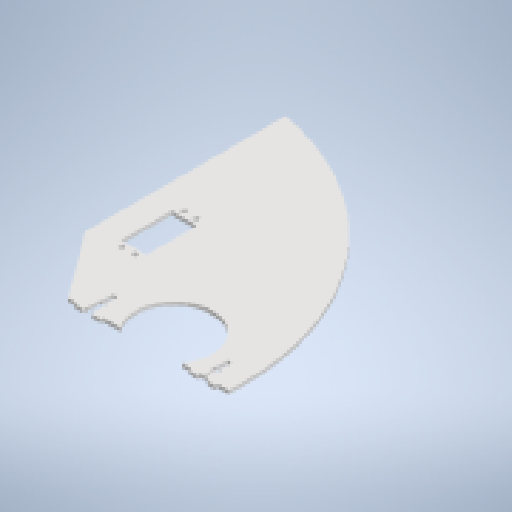
# Autodesk Inventor part: боковые стороны головы
Saved by Autodesk Inventor 2023.2 (Build 272271030, 271C)
## iProperties
Created: 2024-01-31
Part Number: боковые стороны головы
Material: Типовые
Document SubType Name: Modeling
Designer: I9232
Density: 1 g/cm^3
Appearance: По умолчанию
Author: I9232
Autodesk Inventor part; units mm, degrees
ref_plane "YZ Plane" through (0, 0, 0) normal (1, 0, 0) x (0, 1, 0)
ref_plane "XZ Plane" through (0, 0, 0) normal (0, 1, 0) x (-1, 0, 0)
ref_plane "XY Plane" through (0, 0, 0) normal (0, 0, 1) x (1, 0, 0)
sketch "Эскиз1" plane through (0, 0, 0) normal (0, 1, 0) x (-1, 0, 0)
  line L0 (-165, -96.7538) -> (-38.405, -96.7538)
  line L1 (0, -148.7467) -> (0, -306.7538)
  arc A0 (-165, -96.7538) -> (0, -306.7538) centre (36.5744, -108.1954) ccw
  line L2 (-38.405, -96.7538) -> (0, -148.7467)
  point P0 (0, 0)
  point P1 (-167.673, -110.7197)
  constraints: 6 end point, 2 point on circle, 1 centre point, 1 horizontal, 1 perpendicular
extrude "Выдавливание2" add sketch "Эскиз1" along normal blind 3
sketch "Эскиз3" plane through (0, 0, 0) normal (0, -1, 0) x (1, 0, 0)
  circle A0 centre (100.2049, -111.9664) radius 30
  point P0 (0, 0)
  constraints: 1 centre point
extrude "Выдавливание3" cut sketch "Эскиз3" against normal through all
sketch "Эскиз4" plane through (0, 3, 0) normal (0, 1, 0) x (1, 0, 0)
  line L0 (40.1, 196.7538) -> (20, 196.7538)
  line L1 (20, 196.7538) -> (20, 156.7538)
  line L2 (20, 156.7538) -> (40.1, 156.7538)
  line L3 (40.1, 156.7538) -> (40.1, 196.7538)
  line L4 (40.1, 156.7538) -> (40.1, 149.7538) construction
  line L5 (40.1, 149.7538) -> (30.05, 149.7538) construction
  line L6 (20, 149.7538) -> (20, 156.7538) construction
  line L7 (40.1, 196.7538) -> (40.1, 203.7538) construction
  line L8 (40.1, 203.7538) -> (20, 203.7538) construction
  line L9 (20, 203.7538) -> (20, 196.7538) construction
  line L10 (30.05, 203.7538) -> (30.05, 196.7538) construction
  line L11 (30.05, 156.7538) -> (30.05, 149.7538) construction
  line L12 (30.05, 149.7538) -> (20, 149.7538) construction
  line L13 (35.075, 149.7538) -> (35.075, 156.7538) construction
  line L14 (25.025, 149.7538) -> (25.025, 156.7538) construction
  circle A0 centre (35.075, 152.4038) radius 2.15
  circle A1 centre (25.025, 152.4038) radius 2.15
  line L15 (40.1, 176.7538) -> (20, 176.7538) construction
  circle A2 centre (35.075, 201.1038) radius 2.15
  circle A3 centre (25.025, 201.1038) radius 2.15
  line L16 (0, 306.7538) -> (0, 148.7467) projected
  line L17 (35.075, 201.1038) -> (35.075, 196.7538) construction
  line L18 (25.025, 201.1038) -> (25.025, 196.7538) construction
  line L19 (0, 96.7538) -> (74.348, 96.7538) projected
  point P0 (0, 0)
  dimension "d9" = 20.1
  dimension "d10" = 40
  dimension "d11" = 7
  dimension "d12" = 7
  dimension "d13" = 4.3
  dimension "d14" = 4.3
  dimension "d15" = 4.35
  dimension "d16" = 4.35
  dimension "d37" = 20
  dimension "d38" = 60
  constraints: 36 end point, 11 perpendicular, 7 midpoint, 6 point on line, 4 centre point, 2 parallel, 2 symmetric about line, 1 horizontal, 1 vertical, 2 other
  measures "d9" distance of L1.end L2.end
  measures "d10" distance of L0.end L1.end
  measures "d11" distance of L2.end L4.end
  measures "d12" distance of L0.start L7.end
  measures "d13" diameter of A0
  measures "d14" diameter of A1
  measures "d15" distance of L13.end A0.centre
  measures "d16" distance of A1.centre L14.end
  measures "d37" distance between parallel lines of L16 L1
  measures "d38" distance from line of L19 L11.start
extrude "Выдавливание4" cut sketch "Эскиз4" against normal blind 10
sketch "Эскиз6" plane through (165, 0, -96.7538) normal (0, 0, 1) x (1, 0, 0)
  line L0 (-38.9382, 3) -> (-90.652, 3) construction
  line L1 (-7.5, 3) -> (-14.5, 3)
  line L2 (-14.5, 3) -> (-14.5, 0)
  line L3 (-14.5, 0) -> (-7.5, 0)
  line L4 (-7.5, 0) -> (-7.5, 3)
  line L5 (-21.5, 3) -> (-28.5, 3)
  line L6 (-28.5, 3) -> (-28.5, 0)
  line L7 (-28.5, 0) -> (-21.5, 0)
  line L8 (-21.5, 0) -> (-21.5, 3)
  line L9 (-100, 3) -> (-107, 3)
  line L10 (-107, 3) -> (-107, 0)
  line L11 (-107, 0) -> (-100, 0)
  line L12 (-100, 0) -> (-100, 3)
  line L13 (-114, 3) -> (-121, 3)
  line L14 (-121, 3) -> (-121, 0)
  line L15 (-121, 0) -> (-114, 0)
  line L16 (-114, 0) -> (-114, 3)
  line L17 (-165, 0) -> (-90.652, 0) projected
  line L18 (0, 0) -> (0, 3) projected
  line L19 (-165, 0) -> (-165, 3) projected
  point P0 (-21.5, 1.5)
  point P1 (-14.5, 1.5)
  point P2 (-122.3404, 3.4597)
  point P3 (-114, 1.5)
  point P4 (-107, 1.5)
  point P5 (-103.5, 0)
  point P6 (-117.5, 0)
  point P7 (0, 1.5)
  point P8 (-165, 1.5)
  dimension "d20" = 7
  dimension "d21" = 7
  dimension "d22" = 3
  dimension "d23" = 7
  dimension "d24" = 7
  dimension "d25" = 7
  dimension "d26" = 3
  dimension "d27" = 7
  dimension "d28" = 3
  dimension "d49" = 7.5
  dimension "d50" = 44
  constraints: 32 end point, 8 midpoint, 8 parallel, 4 horizontal, 4 perpendicular, 4 point on line
  measures "d20" distance of L2.end L3.end
  measures "d21" distance of L6.end L7.end
  measures "d22" distance of L7.end L5.start
  measures "d23" distance of point (-21.5, 1.5) point (-14.5, 1.5)
  measures "d24" distance of L10.end L11.end
  measures "d25" distance of L14.end L15.end
  measures "d26" distance of L15.end L13.start
  measures "d27" distance of point (-114, 1.5) point (-107, 1.5)
  measures "d28" distance of L11.end L9.start
  measures "d49" distance from line of L4 point (0, 1.5)
  measures "d50" distance from line of point (-165, 1.5) L14
extrude "Выдавливание5" add sketch "Эскиз6" along normal blind 2
sketch "Эскиз7" plane through (0, 0, 0) normal (0, -1, 0) x (1, 0, 0)
  line L0 (51, -96.7538) -> (58, -96.7538) projected
  line L1 (58, -96.7538) -> (51, -96.7538)
  line L2 (54.5, -96.7538) -> (56.25, -96.7538)
  line L3 (56.25, -116.7538) -> (54.5, -116.7538)
  line L4 (54.5, -116.7538) -> (54.5, -96.7538) construction
  line L5 (52.75, -116.7538) -> (54.5, -116.7538)
  line L6 (51.45, -104.8538) -> (51.45, -107.3538)
  line L7 (57.55, -107.3538) -> (57.55, -104.8538)
  line L8 (57.55, -104.8538) -> (51.45, -107.3538) construction
  line L9 (51.45, -104.8538) -> (57.55, -107.3538) construction
  line L10 (54.5, -104.8538) -> (54.5, -106.1038)
  line L11 (145.0889, -96.7538) -> (148.9111, -96.7538)
  line L12 (148.9111, -96.7538) -> (145.0889, -96.7538)
  line L13 (147, -96.7538) -> (145.25, -96.7538)
  line L14 (148.75, -116.7538) -> (147, -116.7538)
  line L15 (147, -116.7538) -> (147, -96.7538) construction
  line L16 (145.25, -116.7538) -> (147, -116.7538)
  line L17 (143.95, -104.8538) -> (143.95, -107.3538)
  line L18 (150.05, -107.3538) -> (150.05, -104.8538)
  line L19 (150.05, -104.8538) -> (143.95, -107.3538) construction
  line L20 (143.95, -104.8538) -> (150.05, -107.3538) construction
  line L21 (147, -104.8538) -> (147, -106.1038)
  line L22 (143.5, -96.7538) -> (150.5, -96.7538) projected
  line L23 (150.05, -104.8538) -> (148.75, -104.8538)
  line L24 (145.25, -104.8538) -> (143.95, -104.8538)
  line L25 (145.25, -96.7538) -> (145.25, -104.8538)
  line L26 (148.75, -107.3538) -> (148.75, -116.7538)
  line L27 (143.95, -107.3538) -> (145.25, -107.3538)
  line L28 (148.75, -107.3538) -> (150.05, -107.3538)
  line L29 (148.75, -96.7538) -> (148.75, -104.8538)
  line L30 (145.25, -107.3538) -> (145.25, -116.7538)
  line L31 (57.55, -104.8538) -> (56.25, -104.8538)
  line L32 (52.75, -104.8538) -> (51.45, -104.8538)
  line L33 (51.45, -107.3538) -> (52.75, -107.3538)
  line L34 (56.25, -107.3538) -> (57.55, -107.3538)
  line L35 (56.25, -96.7538) -> (56.25, -104.8538)
  line L36 (56.25, -107.3538) -> (56.25, -116.7538)
  line L37 (52.75, -96.7538) -> (52.75, -104.8538)
  line L38 (52.75, -107.3538) -> (52.75, -116.7538)
  line L39 (148.75, -96.7538) -> (145.25, -96.7538)
  point P0 (0, 0)
  point P1 (148.75, -96.7538)
  point P2 (148.75, -104.8538)
  dimension "d31" = 20
  dimension "d32" = 3.5
  dimension "d33" = 6.1
  dimension "d34" = 2.5
  dimension "d43" = 8.1
  dimension "d45" = 3.5
  dimension "d46" = 6.1
  dimension "d47" = 2.5
  dimension "d48" = 8.1
  dimension "d51" = 3.5
  dimension "d52" = 3.5
  dimension "d54" = 20
  constraints: 76 end point, 16 parallel, 10 perpendicular, 7 midpoint, 6 horizontal, 5 collinear, 4 symmetric about line, 1 point on line
  measures "d31" distance of L2.end L3.start
  measures "d32" distance of L5.start L3.start
  measures "d33" distance of L6.end L7.start
  measures "d34" distance of L6.start L6.end
  measures "d43" distance of point (54.5, -96.754) L10.start
  measures "d45" distance of L16.start L14.start
  measures "d46" distance of L17.end L18.start
  measures "d47" distance of L17.start L17.end
  measures "d48" distance of L21.start point (147, -96.754)
  measures "d51" distance between parallel lines of L35 L37
  measures "d52" distance between parallel lines of L25 L29
  measures "d54" distance between parallel lines of L22 L14
extrude "Выдавливание6" cut sketch "Эскиз7" against normal blind 3
